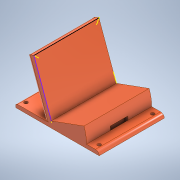
# Autodesk Inventor part: camera mount
Saved by Autodesk Inventor 2020 (Build 240168000, 168)
## iProperties
Created: 2019-06-04
Part Number: camera mount
Material: Generic
Document SubType Name: Modeling
Designer: kangh
Density: 1 g/cm^3
Appearance: Smooth - Light Orange
Author: kangh
## iProperties of the stored document _3DPrint.ipt
Created: 2019-06-04
Part Number: _3DPrint
Material: Generic
Document SubType Name: Modeling
Designer: kangh
Density: 1 g/cm^3
Appearance: Default
Author: kangh
Autodesk Inventor part; units mm, degrees
ref_plane "YZ Plane" through (0, 0, 0) normal (1, 0, 0) x (0, 1, 0)
ref_plane "XZ Plane" through (0, 0, 0) normal (0, 1, 0) x (-1, 0, 0)
ref_plane "XY Plane" through (0, 0, 0) normal (0, 0, 1) x (1, 0, 0)
sketch "Sketch1" plane through (0, 0, 0) normal (0, 1, 0) x (-1, 0, 0)
  line L0 (0, 0) -> (0, 28)
  line L1 (0, 28) -> (0, 23)
  circle A0 centre (5, 23) radius 1.5
  circle A1 centre (68, 23) radius 1.5
  line L2 (0, 28) -> (71.7701, 28)
  line L3 (71.7701, 28) -> (71.7701, 0)
  line L4 (71.7701, 0) -> (0, 0)
  line L5 (0, 0) -> (0, -28)
  line L6 (0, -28) -> (0, -23)
  line L7 (0, -23) -> (5, -23)
  circle A2 centre (5, -23) radius 1.5
  circle A3 centre (68, -23) radius 1.5
  line L8 (0, -28) -> (71.7701, -28)
  line L9 (71.7701, -28) -> (71.7701, 0)
  dimension "d0" = 28
  dimension "d4" = 3
  dimension "d6" = 3
  constraints: 20 end point, 5 symmetric about line, 4 centre point, 2 point on line, 1 coincident, 1 horizontal, 1 perpendicular, 1 vertical, 2 other
  measures "d0" distance of L0.start L0.end
  measures "d4" diameter of A0
  measures "d6" diameter of A1
extrude "Extrusion1" add sketch "Sketch1" along normal blind 3.175
sketch "Sketch2" plane through (0, 3.175, 0) normal (0, 1, 0) x (1, 0, 0)
  line L0 (0, 28) -> (-71.7701, 28) projected
  line L1 (-10.8543, 28) -> (-10.8543, -28)
  line L2 (-71.7701, -28) -> (0, -28) projected
  line L3 (-10.8543, -28) -> (-40.8543, -28)
  line L4 (-40.8543, -28) -> (-40.8543, 28)
  line L5 (-40.8543, 28) -> (-10.8543, 28)
  line L6 (-40.8543, -28) -> (-47.2043, -28)
  line L7 (-47.2043, -28) -> (-47.2043, 28)
  line L8 (-40.8543, 28) -> (-47.2043, 28)
  point P0 (0, 0)
  dimension "d9" = 30
  dimension "d10" = 6.35
  constraints: 14 end point, 6 point on line, 3 perpendicular, 1 collinear, 1 vertical
  measures "d9" distance of L1.end L3.end
  measures "d10" distance of L3.end L6.end
revolve "Revolution1" add sketch "Sketch2" angle 20 about axis through (-47.2043, 3.175, 28) along (0, 0, 1)
sketch "Sketch3" plane through (-47.2043, 3.175, 28) normal (-0.342, 0.9397, 0) x (0.9397, 0.342, 0)
  line L0 (0, 0) -> (0, 56) projected
  line L1 (0, 56) -> (6.35, 56)
  line L2 (43.2716, 56) -> (-24.1703, 56) projected
  line L3 (6.35, 56) -> (6.35, 0)
  line L4 (0, 0) -> (36.35, 0) projected
  line L5 (-23.0843, 0) -> (0, 0) projected
  line L6 (6.35, 0) -> (0, 0)
  line L7 (0, 0) -> (0, 56)
  point P0 (43.2716, 28)
  dimension "d12" = 6.35
  constraints: 8 end point, 2 perpendicular, 2 point on line, 1 horizontal
  measures "d12" distance of L0.end L1.end
extrude "Extrusion2" add sketch "Sketch3" along normal blind 44
sketch "Sketch4" plane through (0, 3.175, 0) normal (0, 1, 0) x (1, 0, 0)
  line L0 (-10.8543, 28) -> (-10.8543, -28) projected
  line L1 (-10.8543, 0) -> (-10.8543, -7.5)
  line L2 (-10.8543, -7.5) -> (-13.8543, -7.5)
  line L3 (-13.8543, -7.5) -> (-13.8543, 0)
  line L4 (-13.8543, 0) -> (-13.8543, 7.5)
  line L5 (-13.8543, 7.5) -> (-10.8543, 7.5)
  line L6 (-10.8543, 7.5) -> (-10.8543, 0)
  point P0 (0, 0)
  dimension "d15" = 7.5
  dimension "d16" = 3
  dimension "d17" = 7.5
  constraints: 12 end point, 4 perpendicular, 3 point on line, 1 midpoint
  measures "d15" distance of L1.start L1.end
  measures "d16" distance of L1.end L2.end
  measures "d17" distance of L3.end L4.end
extrude "Extrusion3" cut sketch "Sketch4" along normal mid plane 6.35
sketch "Sketch5" plane through (0, 3.175, 0) normal (0, 1, 0) x (1, 0, 0)
  line L0 (0, 28) -> (-10.8543, 28) projected
  line L1 (0, 28) -> (-53, 28)
  line L2 (0, 28) -> (-71.7701, 28) projected
  line L3 (-53, 0) -> (-53, 7.5)
  line L4 (-53, 7.5) -> (-56, 7.5)
  line L5 (-56, 7.5) -> (-56, 0)
  line L6 (-56, 0) -> (-56, -7.5)
  line L7 (-56, -7.5) -> (-53, -7.5)
  line L8 (-53, -7.5) -> (-53, 0)
  point P0 (0, 0)
  dimension "d20" = 53
  dimension "d21" = 7.5
  dimension "d22" = 3
  dimension "d23" = 7.5
  constraints: 14 end point, 4 perpendicular, 3 point on line, 1 vertical
  measures "d20" distance of L0.start L1.end
  measures "d21" distance of L3.start L3.end
  measures "d22" distance of L3.end L4.end
  measures "d23" distance of L5.end L6.end
extrude "Extrusion4" cut sketch "Sketch5" against normal blind 6.35
fillet "Fillet1" radius 3.175 8 edges at (0, 3.175, 0) (-54.7287, 23.8482, 28) (-54.7287, 23.8482, -28) (-62.2532, 44.5215, 0) (-56, 3.175, 0) (-53, 3.175, 0) (-54.5, 3.175, -7.5) (-54.5, 3.175, 7.5)
fillet "Fillet2" radius 1.524 1 edges at (-71.7701, 3.175, 0)
sketch "Sketch6" plane through (-41.2373, 5.3468, 28) normal (0.9397, 0.342, 0) x (0, 0, -1)
  line L0 (0, 44) -> (3.175, 40.825) projected
  line L1 (52.825, 40.825) -> (56, 44) projected
  line L2 (0, 44) -> (56, 44)
  point P0 (28, -19.1283)
  constraints: 2 end point, 1 horizontal
sketch "Sketch7" plane through (-41.2373, 5.3468, 28) normal (0.9397, 0.342, 0) x (0, 0, -1)
  line L0 (0, -1.1556) -> (0, 44) projected
  line L1 (0, 0) -> (0, 44)
  line L2 (56, -1.1556) -> (56, 7.8808) projected
  point P0 (28, -19.1283)
  point P1 (56, 44)
  constraints: 2 end point
body "Solid1"
